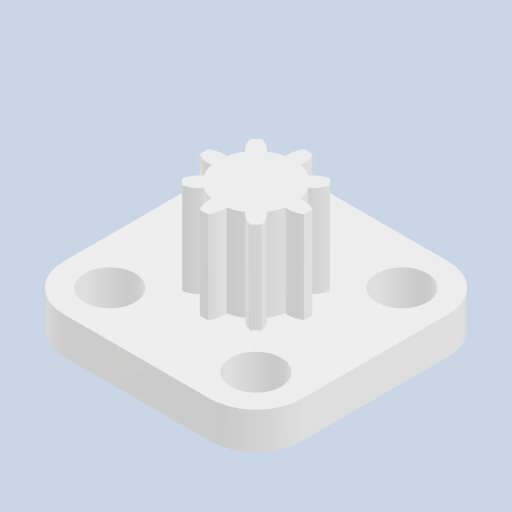
# Autodesk Inventor part: Carrier_V2_CPY
Saved by Autodesk Inventor 2024 (Build 280153000, 153)
## iProperties
Created: 2023-12-13
Part Number: Carrier_V2_CPY
Material: Polystyrene
Document SubType Name: Modeling
Designer: mirun
Density: 1.021 g/cm^3
Appearance: Smooth - White
Author: mirun
Autodesk Inventor part; units mm, degrees
ref_plane "YZ Plane" through (0, 0, 0) normal (1, 0, 0) x (0, 1, 0)
ref_plane "XZ Plane" through (0, 0, 0) normal (0, 1, 0) x (-1, 0, 0)
ref_plane "XY Plane" through (0, 0, 0) normal (0, 0, 1) x (1, 0, 0)
sketch "Sketch1" plane through (0, 0, 0) normal (0, 1, 0) x (-1, 0, 0)
  line L0 (7.955, -7.955) -> (-7.955, -7.955)
  line L1 (-7.955, -7.955) -> (-7.955, 7.955)
  line L2 (-7.955, 7.955) -> (7.955, 7.955)
  line L3 (7.955, 7.955) -> (7.955, -7.955)
  circle A0 centre (7.955, -7.955) radius 5
  circle A1 centre (7.955, -7.955) radius 2.75
  line L4 (0, 0) -> (4.4409, 0)
  line L5 (0, 0) -> (0, 4.5835)
  circle A2 centre (7.955, 7.955) radius 5
  circle A3 centre (7.955, 7.955) radius 2.75
  circle A4 centre (-7.955, -7.955) radius 5
  circle A5 centre (-7.955, -7.955) radius 2.75
  circle A6 centre (-7.955, 7.955) radius 2.75
  circle A7 centre (-7.955, 7.955) radius 5
  line L6 (12.955, 7.955) -> (12.955, -7.955)
  line L7 (7.955, -12.955) -> (-7.955, -12.955)
  line L8 (7.955, 12.955) -> (-7.955, 12.955)
  line L9 (-12.955, 7.955) -> (-12.955, -7.955)
  dimension "d0" = 11.25
  dimension "d1" = 10
  dimension "d2" = 5.5
  constraints: 20 end point, 8 centre point, 8 point on circle, 6 coincident, 6 symmetric about line, 6 tangent, 2 horizontal, 2 vertical, 1 parallel, 15 other
  measures "d0" distance of point (0, 0) L0.start
  measures "d1" diameter of A0
  measures "d2" diameter of A1
extrude "Extrusion1" add sketch "Sketch1" along normal blind 4 contours A4 L1 A5 L0 | A4 L1 A7 L2 A2 L3 A0 L0 | L0 A0 L7 A4 | L0 A5 L1 A4 | A0 L3 A1 L0 | L0 A1 L3 A0 | A4 L9 A7 L1 | L3 A2 L6 A0 | A7 L2 A6 L1 | L1 A6 L2 A7 | A2 L2 A3 L3 | L3 A3 L2 A2 | A7 L8 A2 L2
sketch "Sketch2" plane through (0, 4, 0) normal (0, 1, 0) x (1, 0, 0)
  arc A0 (0.45, 5.6822) -> (0, 5.7) centre (0, 0) ccw
  arc A1 (0.7683, 4.9406) -> (0, 5) centre (0, 0) ccw construction
  arc A2 (0.8, 4.0214) -> (0, 4.1002) centre (0, 0) ccw
  line L0 (0.839, 4.2174) -> (0.8, 4.0214)
  arc A3 (0.839, 4.2174) -> (0, 4.3) centre (0, 0) ccw construction
  arc A4 (0.839, 4.2174) -> (0.45, 5.6822) centre (-1.6581, 4.3383) ccw
  line L1 (-0.839, 4.2174) -> (-0.8, 4.0214)
  arc A5 (-0.45, 5.6822) -> (-0.839, 4.2174) centre (1.6581, 4.3383) ccw
  arc A6 (0, 5) -> (0.7683, 4.9406) centre (0, 0) ccw construction
  arc A7 (0, 5.7) -> (0.45, 5.6822) centre (0, 0) ccw
  arc A8 (0, 4.3) -> (0.839, 4.2174) centre (0, 0) ccw construction
  arc A9 (0, 4.1002) -> (0.8, 4.0214) centre (0, 0) ccw
  dimension "d12" = 10
  dimension "d13" = 2.5
  dimension "d14" = 0.7
  dimension "d15" = 0.7
  dimension "d16" = 0.1998
  dimension "d17" = 0.8
  dimension "d18" = 0.45
  constraints: 24 point on circle, 10 centre point, 4 end point, 3 coincident, 1 line through centre
  measures "d12" diameter of A6
  measures "d13" radius of A5
  measures "d14" distance of A1.end A0.end
  measures "d15" distance of A3.end A1.end
  measures "d16" distance of A2.end A3.end
  measures "d17" horizontal distance of L1.end A2.end
  measures "d18" horizontal distance of A5.start A0.end
extrude "Extrusion2" add sketch "Sketch2" along normal blind 10 contours A9 A2
extrude "Extrusion3" add sketch "Sketch2" along normal blind 10 contours A4 L0 A2 A9 L1 A5 A7 A0
pattern_circular "Circular Pattern1" count 8 over 360 about axis through (0, 4, 0) along (0, 1, 0) of "Extrusion2", "Extrusion3"
body "Solid1"
